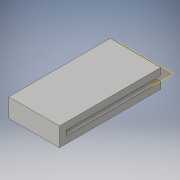
# Autodesk Inventor part: ClipConnector
Saved by Autodesk Inventor 2016 (Build 200138000, 138)
## iProperties
Created: 2016-08-18
Part Number: ClipConnector
Material: Generic
Document SubType Name: Modeling
Designer: yash
Density: 1 g/cm^3
Appearance: Default
Author: yash
Autodesk Inventor part; units mm, degrees
ref_plane "YZ Plane" through (0, 0, 0) normal (1, 0, 0) x (0, 1, 0)
ref_plane "XY Plane" through (0, 0, 0) normal (0, 0, 1) x (1, 0, 0)
sketch "Sketch1" plane through (0, 0, 0) normal (0, 0, 1) x (1, 0, 0)
  line L0 (0, 0) -> (12.7, 0)
  line L1 (12.7, 0) -> (12.7, 1.7272)
  line L2 (12.7, 1.7272) -> (0, 1.7272)
  line L3 (0, 1.7272) -> (0, 0)
  line L4 (0, -1.27) -> (12.7, -1.27)
  line L5 (12.7, -1.27) -> (12.7, -2.9972)
  line L6 (12.7, -2.9972) -> (0, -2.9972)
  line L7 (0, -2.9972) -> (0, -1.27)
  dimension "d0" = 12.7
  dimension "d1" = 1.7272
  dimension "d2" = 12.7
  dimension "d3" = 1.7272
  dimension "d4" = 1.27
  constraints: 16 end point, 4 parallel, 2 horizontal, 2 perpendicular, 1 point on line
  measures "d0" distance of L2.end L1.end
  measures "d1" distance of L1.end L0.end
  measures "d2" distance of L5.end L6.end
  measures "d3" distance of L4.end L5.end
  measures "d4" distance between parallel lines of L0 L4
ref_plane "Work Plane1" through (0, -0.635, 0) normal (0, 1, 0) x (-1, 0, 0)
sketch "Sketch2" plane through (0, -0.635, 0) normal (0, 1, 0) x (-1, 0, 0)
  line L0 (0, 23.6728) -> (-12.7, 23.6728)
  line L1 (-12.7, 23.6728) -> (-12.7, 25.4)
  line L2 (-12.7, 25.4) -> (0, 25.4)
  line L3 (0, 25.4) -> (0, 23.6728)
  point P0 (0, 0)
  point P1 (0, 24.5364)
  dimension "d6" = 12.7
  dimension "d7" = 1.7272
  dimension "d10" = 25.4
  constraints: 8 end point, 2 parallel, 1 horizontal, 1 midpoint, 1 perpendicular, 1 vertical alignment
  measures "d6" distance of L1.end L2.end
  measures "d7" distance of L0.end L1.end
  measures "d10" distance from line of point (0, 0) L2
extrude "Extrusion1" add sketch "Sketch1" along normal blind 25.4
extrude "Extrusion2" add sketch "Sketch2" along normal blind 1.27 and the other way blind 1.27
body "Solid1"
